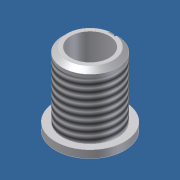
# Autodesk Inventor part: M20ANG2S1M202BR-bushing
Saved by Autodesk Inventor 2014 (Build 180170000, 170)
## iProperties
Category: PARTsolutions
Created: 2013-12-29
Part Number: M20ANG2S1M202BR-bushing
Catalog Web Link: www.cadenas.de
Description: Angle Mount Miniature Toggles - Bushing - Series M - Miniature Toggles
Document SubType Name: Modeling
Designer: PARTsolutions
Material: Generic
Density: 1 g/cm^3
Appearance: RGB(192,192,192)
NB: M20ANG2S1M202BR-bushing
NN: Angle Mount Miniature Toggles - Bushing
NT: Series M - Miniature Toggles
NBSYN: $PN.-bushing
LINA: M20ANG2S1M202BR-bushing
PN: M20ANG2S1M202BR
SRS: M20
PLS: 2
BSHNGALG: 'S1', 'S1 - .350" (8.9mm) Threaded with Keyway','S2', 'S2 - .350" (8.9mm) Smooth with Keyway','A1', 'A1 - .280" (7.1mm) Threaded with Keyway','A2', 'A2 - .280" (7.1mm) Smooth with Keyway','L2', 'L2 - Smooth with Keyway for Lever Lock'
BSHNG: S1
WIDTH: 0.512
HEIGHT: 0.370
LENGTH: 0.500
A: 0.000
TRMNLNOH: 2.000
DMAJ: 0.250
DMIN: 0.219
BSHNGDIA: 0.315
THRDL: 0.350
THRDL2: 0.035
PCDIA: 0.256
PC2: 0.220
PC3: 0.024
KEYPOS: 0.098
KEYW: 0.031
KT: DUMMY
SUPPLIER: NKKSWITCHES
ARTICLENO: M20ANG2S1M202BR-bushing
BOMINFO: M20ANG2S1M202BR-bushing
CREATOR: CADENAS GmbH
PSOL_IDENT_0: {$CADENAS_DATA\23d-libs\nkkswitches\toggle\m\parts\m_ang_t_cover.prj},230 {VTYP=3D},{NB=M20ANG2S1M20
PSOL_IDENT_1: 2BR-bushing},{LINA=M20ANG2S1M202BR-bushing},{NN=Angle Mount Miniature Toggles - Bushing},{DATE=31.05
PSOL_IDENT_2: .2007 10:29:14},{GEOMDATE=31.05.2007 00:00:00},{VERSION=},{LINEID=10},{LINESUBID=-1},{WBVAR=PLS,BSHN
PSOL_IDENT_3: G}  {NB=M20ANG2S1M202BR-bushing},{LINA=M20ANG2S1M202BR-bushing},{KT=DUMMY},{PN=M20ANG2S1M202BR},{SRS
PSOL_IDENT_4: =M20},{PLS=2},{BSHNGALG='S1', 'S1 - .350\" (8.9mm) Threaded with Keyway','S2', 'S2 - .350\" (8.9mm)
PSOL_IDENT_5: Smooth with Keyway','A1', 'A1 - .280\" (7.1mm) Threaded with Keyway','A2', 'A2 - .280\" (7.1mm) Smoo
PSOL_IDENT_6: th with Keyway','L2', 'L2 - Smooth with Keyway for Lever Lock'},{BSHNG=S1},{WIDTH=0.512},{HEIGHT=0.3
PSOL_IDENT_7: 7},{LENGTH=0.5},{A=0},{TRMNLNOH=2},{DMAJ=0.25},{DMIN=0.2193},{BSHNGDIA=0.315},{THRDL=0.35},{THRDL2=0
PSOL_IDENT_8: .035},{PCDIA=0.256},{PC2=0.22},{PC3=0.024},{KEYPOS=0.098},{KEYW=0.031}
Title: M20ANG2S1M202BR-bushing
Author: Cadenas PARTsolutions
Comments: Series M - Miniature Toggles
Autodesk Inventor part; units mm, degrees
sketch "Sketch_1" plane through (0, 0, 0) normal (0, 0, 1) x (1, 0, 0)
  line L0 (-6.35, 0) -> (6.35, 0)
  arc A0 (6.35, 0) -> (6.096, 0.254) centre (6.096, 0) ccw
  line L1 (6.096, 0.254) -> (-6.096, 0.254)
  arc A1 (-6.096, 0.254) -> (-6.35, 0) centre (-6.096, 0) ccw
  constraints: 4 end point, 4 point on circle, 2 centre point
extrude "Extrusion1" add sketch "Sketch_1" along normal mid plane 13.0048
sketch "Sketch_6" plane through (0, 0, 0) normal (0, 0, 1) x (1, 0, 0)
  line L0 (0, 0.127) -> (0, 8.89)
  line L1 (0, 8.89) -> (2.667, 8.89)
  line L2 (2.667, 8.89) -> (3.175, 8.382)
  line L3 (3.175, 8.382) -> (3.175, 1.397)
  line L4 (3.175, 1.397) -> (4.0005, 1.397)
  line L5 (4.0005, 1.397) -> (4.0005, 0.508)
  line L6 (4.0005, 0.508) -> (2.3495, 0.508)
  line L7 (2.3495, 0.508) -> (2.3495, 0.127)
  line L8 (2.3495, 0.127) -> (0, 0.127)
  line L9 (0, 0.127) -> (0, 8.89)
  constraints: 20 end point
revolve "Revolution1" add sketch "Sketch_6" angle 360 about axis through (0, 0.127, 0) along (0, -1, 0)
thread "Thread1" size "1/4-32 UNEF" class "3A" standard "ANSI Unified Screw Threads" length 6.5852 offset 0.3998
sketch "Sketch_8" plane through (0, 0.254, 0) normal (0, 1, 0) x (1, 0, 0)
  line L0 (-0.3937, 2.4892) -> (0.3937, 2.4892)
  line L1 (0.3937, 2.4892) -> (0.3937, 10.4902)
  line L2 (0.3937, 10.4902) -> (-0.3937, 10.4902)
  line L3 (-0.3937, 10.4902) -> (-0.3937, 2.4892)
  constraints: 8 end point
extrude "Extrusion2" cut sketch "Sketch_8" along normal blind 9.779
sketch "Sketch_10_ALT_Drilling_1" plane through (0, 0, 0) normal (0, 0, 1) x (1, 0, 0)
  line L0 (0, 0) -> (0, 9.525)
  line L1 (0, 9.525) -> (2.2225, 9.525)
  line L2 (2.2225, 9.525) -> (2.2225, 0)
  line L3 (2.2225, 0) -> (0, 0)
  line L4 (0, 0) -> (0, 9.525)
  constraints: 10 end point
revolve "Revolution2" cut sketch "Sketch_10_ALT_Drilling_1" angle 360 about axis through (0, 0, 0) along (0, -1, 0)
sketch "Sketch_2" plane through (0, 0, 0) normal (0, 0, 1) x (1, 0, 0)
  line L0 (-6.35, 0.254) -> (-6.35, 0)
  line L1 (-6.35, 0) -> (6.35, 0)
  line L2 (6.35, 0) -> (6.35, 0.254)
  line L3 (6.35, 0.254) -> (-6.35, 0.254)
  constraints: 8 end point
extrude "Extrusion3" cut sketch "Sketch_2" along normal mid plane 13.0048
ref_plane "1_XY" through (0, 7.112, 0) normal (0, 1, 0) x (1, 0, 0)
ref_plane "1_YZ" through (0, 7.112, 0) normal (1, 0, 0) x (0, 0, -1)
ref_plane "1_ZX" through (0, 7.112, 0) normal (0, 0, -1) x (0, 1, 0)
ref_plane "2_XY" through (0, 5.334, 0) normal (0, 1, 0) x (1, 0, 0)
ref_plane "2_YZ" through (0, 5.334, 0) normal (1, 0, 0) x (0, 0, -1)
ref_plane "2_ZX" through (0, 5.334, 0) normal (0, 0, -1) x (0, 1, 0)
ref_plane "3_XY" through (0, 3.556, 0) normal (0, 1, 0) x (1, 0, 0)
ref_plane "3_YZ" through (0, 3.556, 0) normal (1, 0, 0) x (0, 0, -1)
ref_plane "3_ZX" through (0, 3.556, 0) normal (0, 0, -1) x (0, 1, 0)
ref_plane "4_XY" through (0, 2.2225, 0) normal (0, 1, 0) x (1, 0, 0)
ref_plane "4_YZ" through (0, 2.2225, 0) normal (1, 0, 0) x (0, 0, -1)
ref_plane "4_ZX" through (0, 2.2225, 0) normal (0, 0, -1) x (0, 1, 0)
ref_plane "to_base_XY" through (0, 0, 0) normal (0, 1, 0) x (1, 0, 0)
ref_plane "to_base_YZ" through (0, 0, 0) normal (1, 0, 0) x (0, 0, -1)
ref_plane "to_base_ZX" through (0, 0, 0) normal (0, 0, -1) x (0, 1, 0)
body "Solid1"
